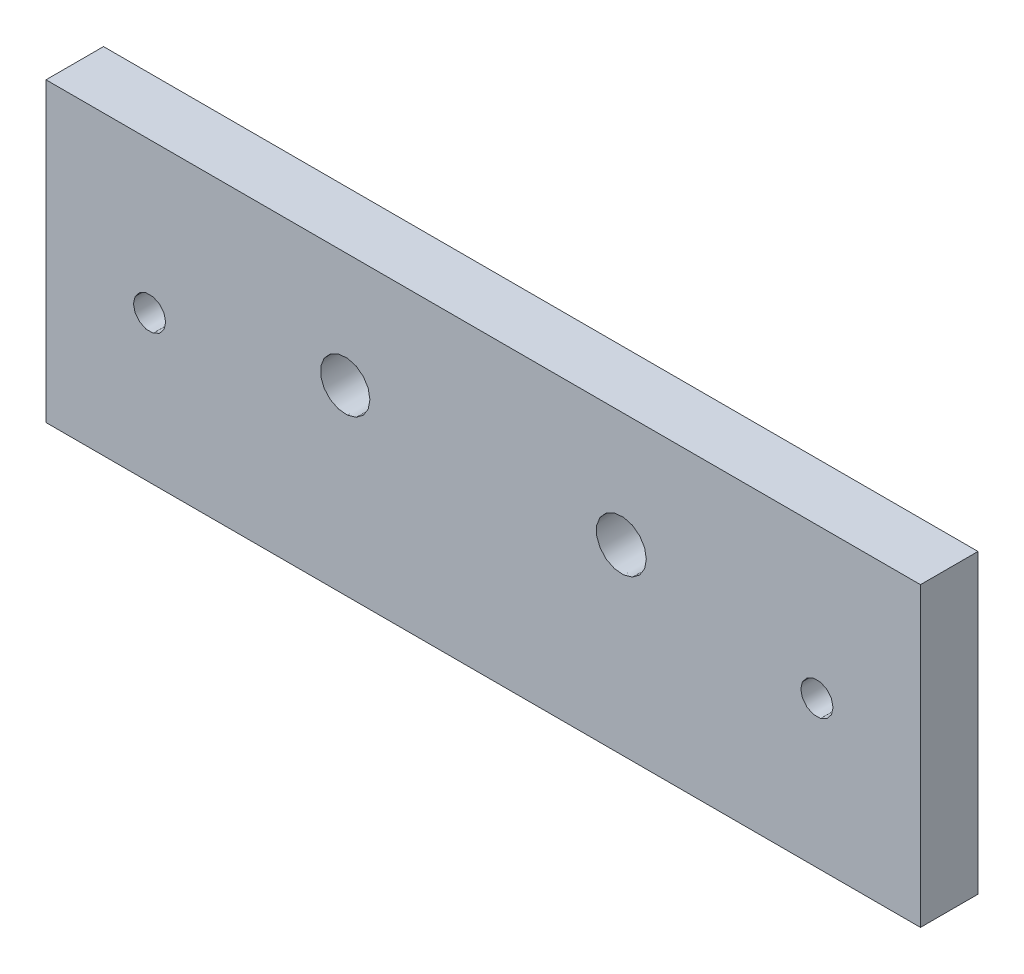
# Autodesk Inventor part: 00_Sandwich_base
Saved by Autodesk Inventor 2024.1 (Build 281209000, 209)
## iProperties
Created: 2024-08-02
Part Number: 00_Sandwich_base
Material: Generisch
Document SubType Name: Modeling
Designer: diederichbenedict
Density: 1 g/cm^3
Appearance: Glatt - Waldgrün
Author: diederichbenedict
Autodesk Inventor part; units mm, degrees
ref_plane "YZ Plane" through (0, 0, 0) normal (1, 0, 0) x (0, 1, 0)
ref_plane "XZ Plane" through (0, 0, 0) normal (0, 1, 0) x (-1, 0, 0)
ref_plane "XY Plane" through (0, 0, 0) normal (0, 0, 1) x (1, 0, 0)
ref_plane "Arbeitsebene1" through (0, 0, 0) normal (0, 0, 1) x (1, 0, 0)
sketch "Skizze1" plane through (0, 0, 0) normal (0, 0, 1) x (1, 0, 0)
  circle A0 centre (-12, 2.9) radius 1.5 projected
  circle A1 centre (12, 2.9) radius 1.5 projected
  line L0 (-38, 12.9) -> (38, 12.9) projected
  line L1 (-38, -12.9) -> (-38, 12.9) projected
  line L2 (38, -12.9) -> (-38, -12.9) projected
  line L3 (38, 12.9) -> (38, -12.9) projected
  circle A2 centre (12, 2.9) radius 2.175
  circle A3 centre (-12, 2.9) radius 2.15
  circle A4 centre (-12, 2.9) radius 1.5 projected
  circle A5 centre (12, 2.9) radius 1.5 projected
  line L4 (-38, 12.9) -> (38, 12.9) projected
  line L5 (-38, -12.9) -> (-38, 12.9) projected
  line L6 (38, -12.9) -> (-38, -12.9) projected
  line L7 (38, 12.9) -> (38, -12.9) projected
  circle A6 centre (29, -0.15) radius 1.6 projected
  circle A7 centre (-29, -0.15) radius 1.6 projected
  circle A8 centre (29, -0.15) radius 1.4
  circle A9 centre (-29, -0.15) radius 1.4
  point P0 (0, 0)
  dimension "d0" = 4.35
  dimension "d1" = 4.3
  dimension "d2" = 2.8
  dimension "d3" = 2.8
  constraints: 4 centre point, 4 coincident
  measures "d0" diameter of A2
  measures "d1" diameter of A3
  measures "d2" diameter of A8
  measures "d3" diameter of A9
extrude "Extrusion1" add sketch "Skizze1" along normal blind 5 contours L0 L3 L2 L1 | A6 | A7
